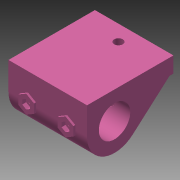
# Autodesk Inventor part: bike_gipper
Saved by Autodesk Inventor 2016 (Build 200138000, 138)
## iProperties
Created: 2015-10-04
Part Number: bike_gipper
Material: Generic
Document SubType Name: Modeling
Designer: eedoga
Density: 1 g/cm^3
Appearance: Pink
Author: eedoga
Autodesk Inventor part; units mm, degrees
ref_plane "YZ Plane" through (0, 0, 0) normal (1, 0, 0) x (0, 1, 0)
sketch "Sketch2" plane through (0, 0, 0) normal (1, 0, 0) x (0, 1, 0)
  circle A0 centre (0, 0) radius 25.4
  arc A1 (0, 44.45) -> (0, -44.45) centre (0, 0) ccw
  line L0 (0, -44.45) -> (0, 25.4)
  line L1 (0, 44.45) -> (44.45, 44.45)
  line L2 (44.45, 44.45) -> (44.45, -44.45)
  line L3 (44.45, -44.45) -> (0, -44.45)
  dimension "d0" = 50.8
  dimension "d2" = 88.9
  dimension "d3" = 44.45
  constraints: 8 end point, 2 coincident, 2 parallel, 2 point on circle, 1 centre point, 1 perpendicular, 1 vertical, 1 vertical alignment, 2 other
  measures "d2" diameter of A1
  measures "d3" distance of L1.start L1.end
extrude "Extrusion1" add sketch "Sketch2" along normal blind 127
sketch "Sketch3" plane through (0, 0, 44.45) normal (0, 0, 1) x (1, 0, 0)
  line L0 (0, 0) -> (127, 0) projected
  line L1 (0, 0) -> (127, 0)
  line L2 (63.5, 0) -> (0, 0)
  line L3 (63.5, 0) -> (127, 0)
  circle A0 centre (31.75, 0) radius 4.2333
  circle A1 centre (95.25, 0) radius 4.2333
  dimension "d6" = 8.4667
  dimension "d7" = 8.4667
  constraints: 6 end point, 3 collinear, 3 midpoint, 2 centre point
  measures "d6" diameter of A0
  measures "d7" diameter of A1
hole "Hole1" at (95.25, 0, 44.45) at (31.75, 0, 44.45) direction (0, 0, -1) diameter 6.35 end through all
ref_plane "Work Plane1" through (0, 0, -25.4) normal (0, 0, -1) x (-1, 0, 0)
sketch "Sketch4" plane through (0, 0, -25.4) normal (0, 0, -1) x (-1, 0, 0)
  arc A0 (-92.075, 0) -> (-98.425, 0) centre (-95.25, 0) ccw projected
  arc A1 (-28.575, 0) -> (-34.925, 0) centre (-31.75, 0) ccw projected
  line L0 (-95.25, 0) -> (-101.6, 0)
  line L1 (-101.6, 3.6662) -> (-95.25, 7.3323)
  line L2 (-95.25, 7.3323) -> (-88.9, 3.6662)
  line L3 (-88.9, 3.6662) -> (-88.9, -3.6662)
  line L4 (-88.9, -3.6662) -> (-95.25, -7.3323)
  line L5 (-95.25, -7.3323) -> (-101.6, -3.6662)
  line L6 (-101.6, -3.6662) -> (-101.6, 3.6662)
  line L7 (-31.75, 0) -> (-25.4, 0)
  line L8 (-25.4, -3.6662) -> (-31.75, -7.3323)
  line L9 (-31.75, -7.3323) -> (-38.1, -3.6662)
  line L10 (-38.1, -3.6662) -> (-38.1, 3.6662)
  line L11 (-38.1, 3.6662) -> (-31.75, 7.3323)
  line L12 (-31.75, 7.3323) -> (-25.4, 3.6662)
  line L13 (-25.4, 3.6662) -> (-25.4, -3.6662)
  point P0 (0, 0)
  dimension "d15" = 6.35
  constraints: 28 end point, 2 coincident, 2 midpoint, 1 horizontal, 1 perpendicular, 26 other
  measures "d15" distance of L0.start L0.end
extrude "Extrusion2" add sketch "Sketch4" along normal blind 6.35
extrude "Extrusion3" cut sketch "Sketch4" against normal blind 57.15
sketch "Sketch5" plane through (0, 0, -44.45) normal (0, 0, -1) x (-1, 0, 0)
  line L0 (-101.6, 3.6662) -> (-95.25, 7.3323) projected
  line L1 (-95.25, 7.3323) -> (-88.9, 3.6662) projected
  line L2 (-88.9, 3.6662) -> (-88.9, -3.6662) projected
  line L3 (-34.925, 0) -> (-92.075, 0) projected
  line L4 (0, 0) -> (-28.575, 0) projected
  line L5 (0, 0) -> (0, 0) projected
  line L6 (0, 0) -> (-28.575, 0) projected
  line L7 (-34.925, 0) -> (-92.075, 0) projected
  line L8 (-98.425, 0) -> (-127, 0) projected
  line L9 (-127, 0) -> (-127, 0) projected
  line L10 (-98.425, 0) -> (-127, 0) projected
  line L11 (-88.9, -3.6662) -> (-95.25, -7.3323) projected
  line L12 (-95.25, -7.3323) -> (-101.6, -3.6662) projected
  line L13 (-101.6, -3.6662) -> (-101.6, 3.6662) projected
  line L14 (-38.1, 3.6662) -> (-31.75, 7.3323) projected
  line L15 (-25.4, -3.6662) -> (-31.75, -7.3323) projected
  line L16 (-31.75, 7.3323) -> (-25.4, 3.6662) projected
  line L17 (-25.4, 3.6662) -> (-25.4, -3.6662) projected
  line L18 (-38.1, -3.6662) -> (-38.1, 3.6662) projected
  line L19 (-31.75, -7.3323) -> (-38.1, -3.6662) projected
  constraints: 4 horizontal alignment
extrude "Extrusion4" cut sketch "Sketch5" against normal blind 3.175
sketch "Sketch6" plane through (0, 0, 44.45) normal (0, 0, 1) x (1, 0, 0)
  line L0 (25.4, 0) -> (25.4, -3.6662) projected
  line L1 (25.4, -3.6662) -> (31.75, -7.3323) projected
  line L2 (31.75, -7.3323) -> (38.1, -3.6662) projected
  line L3 (38.1, -3.6662) -> (38.1, 0) projected
  line L4 (38.1, 0) -> (88.9, 0) projected
  line L5 (88.9, 0) -> (88.9, -3.6662) projected
  line L6 (88.9, -3.6662) -> (95.25, -7.3323) projected
  line L7 (95.25, -7.3323) -> (101.6, -3.6662) projected
  line L8 (101.6, -3.6662) -> (101.6, 0) projected
  line L9 (101.6, 0) -> (127, 0) projected
  line L10 (127, 0) -> (127, 0) projected
  line L11 (98.425, 0) -> (127, 0) projected
  line L12 (34.925, 0) -> (92.075, 0) projected
  line L13 (0, 0) -> (28.575, 0) projected
  line L14 (0, 0) -> (0, 0) projected
  line L15 (0, 0) -> (25.4, 0) projected
  line L16 (38.1, 3.6662) -> (31.75, 7.3323) projected
  line L17 (38.1, -3.6662) -> (38.1, 3.6662) projected
  line L18 (31.75, 7.3323) -> (25.4, 3.6662) projected
  line L19 (25.4, 3.6662) -> (25.4, -3.6662) projected
  line L20 (88.9, 3.6662) -> (88.9, -3.6662) projected
  line L21 (95.25, 7.3323) -> (88.9, 3.6662) projected
  line L22 (101.6, 3.6662) -> (95.25, 7.3323) projected
  line L23 (101.6, -3.6662) -> (101.6, 3.6662) projected
  constraints: 2 horizontal alignment
extrude "Extrusion5" cut sketch "Sketch6" against normal blind 3.175
sketch "Sketch7" plane through (0, 0, -44.45) normal (0, 0, -1) x (-1, 0, 0)
  line L0 (-101.6, 0) -> (-127, 0) projected
  line L1 (-101.6, 0) -> (-101.6, 3.6662) projected
  line L2 (-101.6, 3.6662) -> (-95.25, 7.3323) projected
  line L3 (-95.25, 7.3323) -> (-88.9, 3.6662) projected
  line L4 (-88.9, 3.6662) -> (-88.9, 0) projected
  line L5 (-38.1, 0) -> (-88.9, 0) projected
  line L6 (-95.25, 0) -> (-107.95, 0)
  line L7 (-31.75, 0) -> (-44.45, 0)
  line L8 (-107.95, 7.3323) -> (-95.25, 14.6647)
  line L9 (-95.25, 14.6647) -> (-82.55, 7.3323)
  line L10 (-82.55, 7.3323) -> (-82.55, -7.3323)
  line L11 (-82.55, -7.3323) -> (-95.25, -14.6647)
  line L12 (-95.25, -14.6647) -> (-107.95, -7.3323)
  line L13 (-107.95, -7.3323) -> (-107.95, 7.3323)
  line L14 (-44.45, 7.3323) -> (-31.75, 14.6647)
  line L15 (-31.75, 14.6647) -> (-19.05, 7.3323)
  line L16 (-19.05, 7.3323) -> (-19.05, -7.3323)
  line L17 (-19.05, -7.3323) -> (-31.75, -14.6647)
  line L18 (-31.75, -14.6647) -> (-44.45, -7.3323)
  line L19 (-44.45, -7.3323) -> (-44.45, 7.3323)
  line L20 (-95.25, -7.3323) -> (-88.9, -3.6662) projected
  line L21 (-88.9, -3.6662) -> (-88.9, 0) projected
  line L22 (-101.6, -3.6662) -> (-95.25, -7.3323) projected
  line L23 (-101.6, 0) -> (-101.6, -3.6662) projected
  circle A0 centre (-31.75, 0) radius 3.175 projected
  line L24 (-38.1, 3.6662) -> (-31.75, 7.3323) projected
  line L25 (-38.1, -3.6662) -> (-38.1, 3.6662) projected
  line L26 (-31.75, -7.3323) -> (-38.1, -3.6662) projected
  line L27 (-25.4, -3.6662) -> (-31.75, -7.3323) projected
  line L28 (-25.4, 3.6662) -> (-25.4, -3.6662) projected
  line L29 (-31.75, 7.3323) -> (-25.4, 3.6662) projected
  dimension "d24" = 12.7
  dimension "d25" = 12.7
  constraints: 28 end point, 3 point on line, 2 coincident, 2 midpoint, 26 other
  measures "d24" distance of L6.start L6.end
  measures "d25" distance of L7.start L7.end
extrude "Extrusion6" add sketch "Sketch7" along normal mid plane 6.35 contours L23 L22 L20 L21 L5 L10 L11 L12 L13 L0 | L0 L13 L8 L9 L10 L5 L4 L3 L2 L1 | L19 L14 L15 L16 L17 L18
sketch "Sketch8" plane through (0, 0, 44.45) normal (0, 0, 1) x (1, 0, 0)
  line L0 (101.6, 3.6662) -> (95.25, 7.3323) projected
  line L1 (95.25, 7.3323) -> (88.9, 3.6662) projected
  line L2 (88.9, 3.6662) -> (88.9, -3.6662) projected
  line L3 (88.9, -3.6662) -> (95.25, -7.3323) projected
  line L4 (95.25, -7.3323) -> (101.6, -3.6662) projected
  line L5 (101.6, -3.6662) -> (101.6, 3.6662) projected
  line L6 (107.95, 7.3323) -> (107.95, -7.3323) projected
  line L7 (107.95, -7.3323) -> (95.25, -14.6647) projected
  line L8 (95.25, -14.6647) -> (82.55, -7.3323) projected
  line L9 (82.55, -7.3323) -> (82.55, 7.3323) projected
  line L10 (82.55, 7.3323) -> (95.25, 14.6647) projected
  line L11 (95.25, 14.6647) -> (107.95, 7.3323) projected
  line L12 (31.75, 7.3323) -> (25.4, 3.6662) projected
  line L13 (25.4, 3.6662) -> (25.4, -3.6662) projected
  line L14 (25.4, -3.6662) -> (31.75, -7.3323) projected
  line L15 (31.75, -7.3323) -> (38.1, -3.6662) projected
  line L16 (38.1, -3.6662) -> (38.1, 3.6662) projected
  line L17 (38.1, 3.6662) -> (31.75, 7.3323) projected
  line L18 (44.45, 7.3323) -> (44.45, -7.3323) projected
  line L19 (44.45, -7.3323) -> (31.75, -14.6647) projected
  line L20 (31.75, -14.6647) -> (19.05, -7.3323) projected
  line L21 (19.05, -7.3323) -> (19.05, 7.3323) projected
  line L22 (19.05, 7.3323) -> (31.75, 14.6647) projected
  line L23 (31.75, 14.6647) -> (44.45, 7.3323) projected
extrude "Extrusion7" add sketch "Sketch8" along normal mid plane 6.35
sketch "Sketch11" plane through (0, 0, -44.45) normal (0, 0, -1) x (-1, 0, 0)
  line L0 (-107.95, 0) -> (-107.95, 7.3323) projected
  line L1 (-107.95, 7.3323) -> (-95.25, 14.6647) projected
  line L2 (-95.25, 14.6647) -> (-82.55, 7.3323) projected
  line L3 (-82.55, 7.3323) -> (-82.55, 0) projected
  line L4 (-44.45, 0) -> (-82.55, 0) projected
  line L5 (-44.45, 0) -> (-44.45, 7.3323) projected
  line L6 (-44.45, 7.3323) -> (-31.75, 14.6647) projected
  line L7 (-31.75, 14.6647) -> (-19.05, 7.3323) projected
  line L8 (-19.05, 7.3323) -> (-19.05, 0) projected
  line L9 (0, 0) -> (-19.05, 0) projected
  line L10 (0, 0) -> (0, 44.45) projected
  line L11 (0, 44.45) -> (-127, 44.45) projected
  line L12 (-127, 0) -> (-127, 44.45) projected
  line L13 (-107.95, 0) -> (-127, 0) projected
  line L14 (-127, 44.45) -> (0, 44.45)
  line L15 (0, 44.45) -> (0, 19.05)
  line L16 (0, 19.05) -> (-127, 19.05)
  line L17 (-127, 19.05) -> (-127, 44.45)
  constraints: 8 end point, 2 parallel, 1 horizontal, 1 perpendicular, 1 point on line
extrude "Extrusion9" add sketch "Sketch11" along normal blind 50.8 contours L12 L11 L10 L16
ref_plane "Work Plane2" through (63.5, 0, 0) normal (1, 0, 0) x (0, 0, -1)
sketch "Sketch13" plane through (63.5, 0, 0) normal (1, 0, 0) x (0, 0, -1)
  circle A0 centre (0, 0) radius 25.4 projected
  arc A1 (-44.45, 0) -> (44.45, 0) centre (0, 0) ccw projected
  line L0 (44.45, 0) -> (44.45, 19.05) projected
  line L1 (44.45, 19.05) -> (95.25, 19.05) projected
  line L2 (95.25, 44.45) -> (95.25, 19.05) projected
  line L3 (-44.45, 44.45) -> (95.25, 44.45) projected
  line L4 (-44.45, 44.45) -> (-44.45, 0) projected
  line L5 (95.25, 19.05) -> (88.9, 19.05)
  line L6 (88.9, 19.05) -> (29.3739, -33.3613)
  dimension "d65" = 6.35
  constraints: 4 end point, 1 point on circle, 1 point on line, 1 tangent
  measures "d65" distance of L1.end L5.end
extrude "Extrusion10" add sketch "Sketch13" along normal mid plane 25.4 contours A1 L0 L1 L6
sketch "Sketch14" plane through (127, 0, 0) normal (1, 0, 0) x (0, 0, -1)
  arc A0 (29.3739, -33.3613) -> (44.45, 0) centre (0, 0) ccw projected
  line L0 (29.3739, -33.3613) -> (88.9, 19.05) projected
  line L1 (44.45, 19.05) -> (88.9, 19.05) projected
  line L2 (44.45, 0) -> (44.45, 19.05) projected
  circle A1 centre (0, 0) radius 25.4 projected
  arc A2 (-44.45, 0) -> (44.45, 0) centre (0, 0) ccw projected
  line L3 (44.45, 0) -> (44.45, 19.05) projected
  line L4 (44.45, 19.05) -> (95.25, 19.05) projected
  line L5 (95.25, 44.45) -> (95.25, 19.05) projected
  line L6 (-44.45, 44.45) -> (95.25, 44.45) projected
  line L7 (-44.45, 44.45) -> (-44.45, 0) projected
extrude "Extrusion11" add sketch "Sketch14" against normal blind 12.7 contours A0 L2 L1 L0
sketch "Sketch15" plane through (0, 0, 0) normal (-1, 0, 0) x (0, 0, 1)
  arc A0 (-44.45, 0) -> (-29.3739, -33.3613) centre (0, 0) ccw projected
  line L0 (-44.45, 19.05) -> (-44.45, 0) projected
  line L1 (-88.9, 19.05) -> (-44.45, 19.05) projected
  line L2 (-88.9, 19.05) -> (-29.3739, -33.3613) projected
  circle A1 centre (0, 0) radius 25.4 projected
  arc A2 (-44.45, 0) -> (44.45, 0) centre (0, 0) ccw projected
  line L3 (44.45, 44.45) -> (44.45, 0) projected
  line L4 (44.45, 44.45) -> (-95.25, 44.45) projected
  line L5 (-95.25, 19.05) -> (-95.25, 44.45) projected
  line L6 (-44.45, 19.05) -> (-95.25, 19.05) projected
  line L7 (-44.45, 0) -> (-44.45, 19.05) projected
extrude "Extrusion12" add sketch "Sketch15" against normal blind 12.7 contours A0 L2 L1 L0
sketch "Sketch16" plane through (0, 44.45, 44.45) normal (0, 1, 0) x (1, 0, 0)
  line L0 (0, 0) -> (0, 139.7) projected
  line L1 (127, 0) -> (127, 139.7) projected
  line L2 (107.95, 88.9) -> (114.3, 88.9) projected
  line L3 (107.95, 88.9) -> (95.25, 88.9) projected
  line L4 (95.25, 88.9) -> (82.55, 88.9) projected
  line L5 (76.2, 88.9) -> (82.55, 88.9) projected
  line L6 (76.2, 88.9) -> (114.3, 88.9) projected
  line L7 (114.3, 88.9) -> (127, 88.9)
  line L8 (127, 88.9) -> (0, 88.9)
  line L9 (0, 88.9) -> (127, 88.9)
  line L10 (127, 88.9) -> (127, 139.7)
  line L11 (127, 139.7) -> (0, 139.7)
  line L12 (0, 139.7) -> (0, 88.9)
  circle A0 centre (63.5, 114.3) radius 6.985
  point P0 (0, 44.45)
  dimension "d72" = 13.97
  constraints: 12 end point, 3 perpendicular, 2 parallel, 2 point on line, 1 centre point, 1 horizontal
  measures "d72" diameter of A0
hole "Hole3" at (63.5, 44.45, -69.85) direction (0, -1, 0) diameter 13.97 end through all
sketch "Sketch17" plane through (63.5, 0, 0) normal (1, 0, 0) x (0, 0, -1)
  line L0 (62.865, 44.45) -> (76.835, 44.45) projected
  line L1 (62.865, 44.45) -> (43.815, 44.45)
  line L2 (69.85, 44.45) -> (69.85, 57.15)
  line L3 (69.85, 57.15) -> (43.815, 44.45)
  point P0 (0, 0)
  dimension "d81" = 19.05
  dimension "d82" = 12.7
  constraints: 6 end point, 1 collinear, 1 midpoint, 1 perpendicular
  measures "d81" distance of L0.start L1.end
  measures "d82" distance of L2.start L2.end
body "Solid1"
